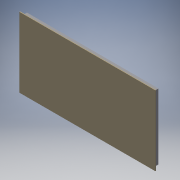
# Autodesk Inventor part: gatorboard_01875in_front_door
Saved by Autodesk Inventor 2019 (Build 230136000, 136)
## iProperties
Created: 2019-03-10
Part Number: gatorboard_01875in_front_door
Material: Generic
Document SubType Name: Modeling
Designer: Wilson Lab
Density: 1 g/cm^3
Appearance: Default
Author: Wilson Lab
Autodesk Inventor part; units mm, degrees
ref_plane "YZ Plane" through (0, 0, 0) normal (1, 0, 0) x (0, 1, 0)
ref_plane "XZ Plane" through (0, 0, 0) normal (0, 1, 0) x (-1, 0, 0)
ref_plane "XY Plane" through (0, 0, 0) normal (0, 0, 1) x (1, 0, 0)
sketch "Sketch1" plane through (0, 0, 0) normal (0, 0, 1) x (1, 0, 0)
  line L0 (0, 0) -> (774.7, 0)
  line L1 (774.7, 0) -> (774.7, 398.78)
  line L2 (774.7, 398.78) -> (0, 398.78)
  line L3 (0, 398.78) -> (0, 0)
  dimension "d2" = 774.7
  dimension "d3" = 398.78
  constraints: 8 end point, 2 parallel, 1 coincident, 1 horizontal, 1 perpendicular
  measures "d2" distance of L1.end L2.end
  measures "d3" distance of L0.end L1.end
extrude "Extrusion1" add sketch "Sketch1" along normal blind 4.7625
sketch "Sketch2" plane through (0, 0, 0) normal (0, 0, -1) x (-1, 0, 0)
  line L0 (-800.6197, 386.715) -> (24.8803, 386.715) projected
  line L1 (-13.2197, 386.715) -> (-13.2197, 12.065) projected
  line L2 (-800.6197, 12.065) -> (24.8803, 12.065) projected
  line L3 (-762.5197, 386.715) -> (-762.5197, 12.065) projected
  line L4 (-13.2197, 12.065) -> (-762.5197, 12.065)
  line L5 (-762.5197, 12.065) -> (-762.5197, 386.715)
  line L6 (-762.5197, 386.715) -> (-13.2197, 386.715)
  line L7 (-13.2197, 386.715) -> (-13.2197, 12.065)
  point P0 (0, 0)
  constraints: 8 end point, 2 parallel, 1 horizontal, 1 perpendicular
extrude "Extrusion2" add sketch "Sketch2" along normal blind 25.4
body "Solid1"
